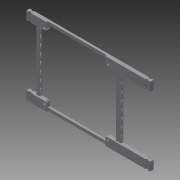
# Autodesk Inventor part: NUCholder
Saved by Autodesk Inventor 2015 (Build 190159000, 159)
## iProperties
Created: 2015-04-17
Part Number: NUCholder
Material: NylonD2W
Document SubType Name: Modeling
Designer: Akovo_000
Density: 0.93 g/cm^3
Appearance: Nylon 6
Mass: 13.1398 g
Surface Area: 149.789 cm^2
Volume: 14.1288 cm^3
Author: Akovo_000
Autodesk Inventor part; units mm, degrees
ref_plane "YZ Plane" through (0, 0, 0) normal (1, 0, 0) x (0, 1, 0)
ref_plane "XZ Plane" through (0, 0, 0) normal (0, 1, 0) x (-1, 0, 0)
ref_plane "XY Plane" through (0, 0, 0) normal (0, 0, 1) x (1, 0, 0)
sketch "Button Layer" plane through (0, 0, 0) normal (0, 1, 0) x (-1, 0, 0)
  line L0 (-73.3766, -28.1226) -> (16.7234, -28.1226)
  circle A0 centre (16.7234, -28.1226) radius 1.5
  circle A1 centre (-73.3766, -28.1226) radius 1.5
  line L1 (16.7234, 2.8734) -> (-73.3766, 2.8734)
  circle A2 centre (-11.2766, 30.8734) radius 28
  line L2 (-73.3766, 2.8734) -> (-73.3766, -28.1226)
  line L3 (-73.3766, 47.3774) -> (-73.3766, 2.8734)
  line L4 (16.7234, 2.8734) -> (16.7234, 58.8734)
  line L5 (16.7234, 2.8734) -> (16.7234, -28.1226)
  circle A3 centre (9.7234, -21.1226) radius 3
  circle A4 centre (9.7234, -21.1226) radius 2.5
  line L6 (9.7234, -21.1226) -> (16.7234, -21.1226)
  line L7 (16.7234, -21.1226) -> (16.7234, -28.1226)
  line L8 (16.7234, -28.1226) -> (9.7234, -28.1226)
  line L9 (9.7234, -28.1226) -> (9.7234, -21.1226)
  line L10 (9.7234, -21.1226) -> (-2.2766, -21.1226)
  line L11 (-2.2766, -21.1226) -> (-2.2766, -15.6226)
  line L12 (-2.2766, -15.6226) -> (9.7234, -15.6226)
  line L13 (9.7234, -15.6226) -> (9.7234, -21.1226)
  circle A5 centre (9.7234, -15.6226) radius 2.5
  circle A6 centre (-2.2766, -15.6226) radius 2.5
  line L14 (15.1646, -25.4226) -> (18.2823, -25.4226)
  line L15 (18.2823, -25.4226) -> (19.8411, -28.1226)
  line L16 (19.8411, -28.1226) -> (18.2823, -30.8226)
  line L17 (18.2823, -30.8226) -> (15.1646, -30.8226)
  line L18 (15.1646, -30.8226) -> (13.6057, -28.1226)
  line L19 (13.6057, -28.1226) -> (15.1646, -25.4226)
  line L20 (-74.9354, -25.4226) -> (-71.8177, -25.4226)
  line L21 (-71.8177, -25.4226) -> (-70.2589, -28.1226)
  line L22 (-70.2589, -28.1226) -> (-71.8177, -30.8226)
  line L23 (-71.8177, -30.8226) -> (-74.9354, -30.8226)
  line L24 (-74.9354, -30.8226) -> (-76.4943, -28.1226)
  line L25 (-76.4943, -28.1226) -> (-74.9354, -25.4226)
  line L26 (16.7234, 79.3734) -> (-73.3766, 79.3734)
  line L27 (-73.3766, -15.6266) -> (16.7234, -15.6266)
  circle A7 centre (16.7234, 79.3734) radius 1.5
  circle A8 centre (16.7234, -15.6266) radius 1.5
  circle A9 centre (-73.3766, -15.6266) radius 1.5
  circle A10 centre (-73.3766, 79.3734) radius 1.5
  line L28 (-73.3766, 59.8734) -> (16.7234, 59.8734)
  line L29 (-73.3766, 3.8734) -> (-73.3766, -15.6266)
  line L30 (-73.3766, 59.8734) -> (-73.3766, 79.3734)
  line L31 (-73.3766, 59.8734) -> (-73.3766, 3.8734)
  line L32 (16.7234, 3.8734) -> (16.7234, 59.8734)
  line L33 (16.7234, 3.8734) -> (16.7234, -15.6266)
  circle A11 centre (9.7234, -8.6266) radius 3
  circle A12 centre (9.7234, -8.6266) radius 2.5
  line L34 (9.7234, -8.6266) -> (16.7234, -8.6266)
  line L35 (16.7234, -8.6266) -> (16.7234, -15.6266)
  line L36 (16.7234, -15.6266) -> (9.7234, -15.6266)
  line L37 (9.7234, -15.6266) -> (9.7234, -8.6266)
  line L38 (9.7234, -8.6266) -> (-2.2766, -8.6266)
  line L39 (-2.2766, -8.6266) -> (-2.2766, -3.1266)
  line L40 (-2.2766, -3.1266) -> (9.7234, -3.1266)
  line L41 (9.7234, -3.1266) -> (9.7234, -8.6266)
  circle A13 centre (9.7234, -3.1266) radius 2.5
  circle A14 centre (-2.2766, -3.1266) radius 2.5
  line L42 (15.1646, -12.9266) -> (18.2823, -12.9266)
  line L43 (18.2823, -12.9266) -> (19.8411, -15.6266)
  line L44 (19.8411, -15.6266) -> (18.2823, -18.3266)
  line L45 (18.2823, -18.3266) -> (15.1646, -18.3266)
  line L46 (15.1646, -18.3266) -> (13.6057, -15.6266)
  line L47 (13.6057, -15.6266) -> (15.1646, -12.9266)
  line L48 (15.1646, 82.0734) -> (18.2823, 82.0734)
  line L49 (18.2823, 82.0734) -> (19.8411, 79.3734)
  line L50 (19.8411, 79.3734) -> (18.2823, 76.6734)
  line L51 (18.2823, 76.6734) -> (15.1646, 76.6734)
  line L52 (15.1646, 76.6734) -> (13.6057, 79.3734)
  line L53 (13.6057, 79.3734) -> (15.1646, 82.0734)
  line L54 (-74.9354, 82.0734) -> (-71.8177, 82.0734)
  line L55 (-71.8177, 82.0734) -> (-70.2589, 79.3734)
  line L56 (-70.2589, 79.3734) -> (-71.8177, 76.6734)
  line L57 (-71.8177, 76.6734) -> (-74.9354, 76.6734)
  line L58 (-74.9354, 76.6734) -> (-76.4943, 79.3734)
  line L59 (-76.4943, 79.3734) -> (-74.9354, 82.0734)
  line L60 (-74.9354, -12.9266) -> (-71.8177, -12.9266)
  line L61 (-71.8177, -12.9266) -> (-70.2589, -15.6266)
  line L62 (-70.2589, -15.6266) -> (-71.8177, -18.3266)
  line L63 (-71.8177, -18.3266) -> (-74.9354, -18.3266)
  line L64 (-74.9354, -18.3266) -> (-76.4943, -15.6266)
  line L65 (-76.4943, -15.6266) -> (-74.9354, -12.9266)
  line L66 (41.6234, -38.1226) -> (-138.3766, -38.1226)
  line L67 (-138.3766, -38.1226) -> (-138.3766, 63.8774)
  line L68 (-138.3766, 63.8774) -> (41.6234, 63.8774)
  line L69 (41.6234, 63.8774) -> (41.6234, -38.1226)
  circle A15 centre (-73.3766, -15.6266) radius 3.5
  circle A16 centre (16.7234, -15.6266) radius 3.5
  circle A17 centre (-73.3766, 79.3734) radius 3.5
  circle A18 centre (16.7234, 79.3734) radius 3.5
  line L70 (41.6234, -38.1226) -> (13.2234, -38.1226)
  line L71 (13.2234, -38.1226) -> (13.2234, -12.1266)
  line L72 (13.2234, -12.1266) -> (41.6234, -12.1266)
  line L73 (41.6234, -12.1266) -> (41.6234, -38.1226)
  line L74 (-138.3766, -38.1226) -> (-69.8766, -38.1226)
  line L75 (-69.8766, -38.1226) -> (-69.8766, -12.1266)
  line L76 (-69.8766, -12.1266) -> (-138.3766, -12.1266)
  line L77 (-138.3766, -12.1266) -> (-138.3766, -38.1226)
  line L78 (16.7234, 59.8734) -> (16.7234, 79.3734)
  point P0 (0, 0)
  point P1 (0, 0)
  point P2 (0, 0)
  dimension "d33" = 90.1
  dimension "d35" = 6
  dimension "d36" = 0.5
  dimension "d37" = 5
  dimension "d38" = 12
  dimension "d39" = 7
  dimension "d40" = 5.4
  dimension "d41" = 3
  dimension "d43" = 90.1
  dimension "d45" = 6
  dimension "d46" = 0.5
  dimension "d47" = 5
  dimension "d48" = 12
  dimension "d49" = 7
  dimension "d50" = 5.4
  dimension "d63" = 180
  dimension "d64" = 102
  dimension "d65" = 65
  dimension "d66" = 24.9
  dimension "d67" = 22.496
  dimension "d68" = 7
  dimension "d69" = 10
  dimension "d70" = 57
  constraints: 158 end point, 20 coincident, 19 centre point, 15 parallel, 10 perpendicular, 9 equal length, 9 horizontal, 8 equal radius, 8 tangent, 5 collinear, 4 vertical, 2 concentric, 78 other
  measures "d33" distance of L0.start L0.end
  measures "d35" diameter of A3
  measures "d36" radial gap between concentric circles of A3 A4
  measures "d37" diameter of A5
  measures "d38" distance between parallel lines of L11 L13
  measures "d39" distance of L6.start L6.end
  measures "d40" distance between parallel lines of L15 L18
  measures "d41" diameter of A7
  measures "d43" distance of L27.start L27.end
  measures "d45" diameter of A11
  measures "d46" radial gap between concentric circles of A11 A12
  measures "d47" diameter of A13
  measures "d48" distance between parallel lines of L39 L41
  measures "d49" distance of L34.start L34.end
  measures "d50" distance between parallel lines of L43 L46
  measures "d63" distance of L67.end L68.end
  measures "d64" distance of L66.end L67.end
  measures "d65" distance between parallel lines of L67 L29
  measures "d66" distance between parallel lines of L69 L32
  measures "d67" distance between parallel lines of L66 L27
  measures "d68" diameter of A15
  measures "d69" distance between parallel lines of L66 L0
  measures "d70" distance between parallel lines of L28 L1
sketch "NucSupport" plane through (0, 0, 0) normal (0, 1, 0) x (-1, 0, 0)
  line L0 (0, 0) -> (-175, 0)
  line L1 (-175, 0) -> (-175, 110)
  line L2 (-175, 110) -> (0, 110)
  line L3 (0, 110) -> (0, 0)
  line L4 (-24.9, 8.5) -> (-115, 8.5)
  line L5 (-115, 8.5) -> (-115, 101.5)
  line L6 (-115, 101.5) -> (-24.9, 101.5)
  line L7 (-24.9, 101.5) -> (-24.9, 8.5)
  line L8 (-24.9, 12) -> (0, 12)
  line L9 (-28.4, 8.5) -> (-28.4, 0)
  line L10 (-24.9, 98) -> (0, 98)
  line L11 (-28.4, 101.5) -> (-28.4, 110)
  line L12 (-111.5, 101.5) -> (-111.5, 110)
  line L13 (-115, 98) -> (-175, 98)
  line L14 (-115, 12) -> (-175, 12)
  line L15 (-111.5, 8.5) -> (-111.5, 0)
  circle A0 centre (-115, 8.5) radius 3.5
  circle A1 centre (-24.9, 8.5) radius 3.5
  circle A2 centre (-115, 101.5) radius 3.5
  circle A3 centre (-24.9, 101.5) radius 3.5
  dimension "d174" = 7
  dimension "d71" = 175
  dimension "d72" = 110
  dimension "d73" = 90.1
  dimension "d74" = 93
  dimension "d75" = 60
  dimension "d176" = 24.9
  dimension "d270" = 12
  constraints: 32 end point, 16 point on line, 9 equal length, 4 coincident, 4 horizontal, 2 horizontal alignment, 2 vertical, 2 vertical alignment, 1 perpendicular, 10 other
  measures "d71" distance of L0.start L0.end
  measures "d72" distance of L0.end L1.end
  measures "d73" distance of L5.end L6.end
  measures "d74" distance of L4.end L5.end
  measures "d75" distance between parallel lines of L1 L5
  measures "d176" distance between parallel lines of L3 L7
  measures "d270" distance between parallel lines of L13 L2
extrude "NucSupportHorizontal" add sketch "NucSupport" along normal blind 2 contours L0 L9 A1 L8 L3 | L0 L1 L14 A0 L15 | A1 L7 L4 | L4 L7 A1 | L10 A3 L11 L2 L3 | A0 L5 L4 | L4 L5 A0 | A3 L6 L7 | L7 L6 A3 | L1 L2 L12 A2 L13 | A2 L6 L5 | L5 L6 A2
sketch "Sketch4" plane through (0, 2, 0) normal (0, 1, 0) x (1, 0, 0)
  arc A0 (28.4, -101.5) -> (24.9, -98) centre (24.9, -101.5) ccw projected
  circle A1 centre (24.9, -101.5) radius 3.5
  arc A2 (115, -98) -> (111.5, -101.5) centre (115, -101.5) ccw projected
  circle A3 centre (115, -101.5) radius 3.5
  arc A4 (111.5, -8.5) -> (115, -12) centre (115, -8.5) ccw projected
  circle A5 centre (115, -8.5) radius 3.5
  arc A6 (24.9, -12) -> (28.4, -8.5) centre (24.9, -8.5) ccw projected
  circle A7 centre (24.9, -8.5) radius 3.5
  constraints: 7 equal radius, 4 centre point, 4 coincident
hole "Holes" at (24.9, 2, 101.5) at (24.9, 2, 8.5) at (115, 2, 8.5) at (115, 2, 101.5) direction (0, -1, 0) diameter 3.5 depth 7
sketch "Sketch6" plane through (0, 2, 0) normal (0, 1, 0) x (1, 0, 0)
  line L0 (0, 0) -> (28.4, 0)
  line L1 (28.4, 0) -> (28.4, -8.5)
  line L2 (28.4, -8.5) -> (28.4, 0) projected
  line L3 (24.9, -12) -> (0, -12)
  line L4 (0, -12) -> (0, 0)
  line L5 (0, 0) -> (0, -12) projected
  line L6 (0, -98) -> (24.9, -98)
  line L7 (24.9, -98) -> (0, -98) projected
  line L8 (0, -110) -> (28.4, -110) projected
  line L9 (28.4, -110) -> (0, -110)
  line L10 (0, -110) -> (0, -98)
  line L11 (111.5, -110) -> (111.5, -101.5)
  arc A0 (115, -98) -> (111.5, -101.5) centre (115, -101.5) ccw projected
  line L12 (115, -98) -> (175, -98)
  line L13 (175, -98) -> (115, -98) projected
  line L14 (175, -98) -> (175, -110)
  line L15 (175, -110) -> (111.5, -110)
  line L16 (111.5, 0) -> (175, 0)
  line L17 (175, 0) -> (111.5, 0) projected
  line L18 (175, 0) -> (175, -12)
  line L19 (175, -12) -> (115, -12)
  arc A1 (111.5, -8.5) -> (115, -12) centre (115, -8.5) ccw projected
  line L20 (111.5, -8.5) -> (111.5, 0)
  circle A2 centre (115, -101.5) radius 1.75 projected
  arc A3 (115, -98) -> (111.5, -101.5) centre (115, -101.5) ccw
  circle A4 centre (24.9, -8.5) radius 1.75 projected
  arc A5 (24.9, -12) -> (28.4, -8.5) centre (24.9, -8.5) ccw
  circle A6 centre (115, -8.5) radius 1.75 projected
  arc A7 (111.5, -8.5) -> (115, -12) centre (115, -8.5) ccw
  circle A8 centre (24.9, -101.5) radius 1.75 projected
  arc A9 (28.4, -101.5) -> (24.9, -98) centre (24.9, -101.5) ccw
  arc A10 (28.4, -101.5) -> (24.9, -98) centre (24.9, -101.5) ccw projected
  line L21 (28.4, -101.5) -> (28.4, -110)
  line L22 (0, -12) -> (24.9, -12) projected
  line L23 (28.4, -110) -> (28.4, -101.5) projected
  line L24 (111.5, -101.5) -> (111.5, -110) projected
  line L25 (111.5, 0) -> (111.5, -8.5) projected
  line L26 (16.9, -12) -> (16.9, -98)
  line L27 (11.9, -98) -> (11.9, -12)
  line L28 (125, -12) -> (125, -98)
  line L29 (175, -98) -> (115, -98) projected
  line L30 (115, -12) -> (175, -12) projected
  line L31 (132, -12) -> (132, -98)
  line L32 (28.4, 0) -> (111.5, 0)
  line L33 (111.5, 0) -> (111.5, -4.25)
  line L34 (111.5, -4.25) -> (28.4, -4.25)
  line L35 (28.4, -4.25) -> (28.4, 0)
  line L36 (111.5, -110) -> (28.4, -110)
  line L37 (28.4, -110) -> (28.4, -105.75)
  line L38 (28.4, -105.75) -> (111.5, -105.75)
  line L39 (111.5, -105.75) -> (111.5, -110)
  dimension "d179" = 5
  dimension "d181" = 7
  dimension "d183" = 8
  dimension "d184" = 10
  dimension "d269" = 12
  constraints: 56 end point, 9 perpendicular, 9 point on line, 8 point on circle, 7 parallel, 6 collinear, 5 tangent, 4 centre point, 4 coincident, 3 horizontal, 2 midpoint, 1 vertical
  measures "d179" distance between parallel lines of L27 L26
  measures "d181" distance between parallel lines of L31 L28
  measures "d183" distance from line of L26 A5.centre
  measures "d184" distance from line of A7.centre L28
  measures "d269" distance of L16.end L18.end
extrude "Big Holder" add sketch "Sketch6" along normal blind 3 contours L0 L1 A5 L3 L4 | L32 L20 L34 L1 | L16 L18 L19 A1 L20 | L3 L26 L6 L27 | L6 A9 L21 L8 L10 | L31 L12 L28 L19 | L12 L14 L15 L11 A0 | L21 L38 L11 L36
sketch "Air Grill" plane through (132, 2, 98) normal (1, 0, 0) x (0, 0, -1)
  line L0 (0, 3) -> (86, 3)
  line L1 (86, 3) -> (86, 0)
  line L2 (0, 0) -> (0, 3)
  line L3 (1, 3) -> (85, 3)
  line L4 (85, 3) -> (85, 2.5)
  line L5 (1, 2.5) -> (1, 3)
  line L6 (85, 0) -> (85, 0.5)
  line L7 (1, -1.5) -> (1, -2)
  line L8 (89.5, 3) -> (86, 3) projected
  line L9 (1, 2.5) -> (1, -1.5)
  line L10 (85, 2.5) -> (85, 0.5)
  line L11 (86, 0) -> (86, 3) projected
  line L12 (1, 2.5) -> (5.5566, 0.5)
  line L13 (1, 2.5) -> (5.9762, 2.5) construction
  line L14 (7.2983, 0.5) -> (10.0583, 2.5)
  line L15 (7.2983, 0.5) -> (10.7067, 0.5) construction
  line L16 (11.8, 2.5) -> (16.3566, 0.5)
  line L17 (18.0982, 0.5) -> (20.8583, 2.5)
  line L18 (18.0982, 0.5) -> (21.5067, 0.5) construction
  line L19 (22.5999, 2.5) -> (27.1565, 0.5)
  line L20 (28.8982, 0.5) -> (31.6582, 2.5)
  line L21 (28.8982, 0.5) -> (32.3067, 0.5) construction
  line L22 (33.3999, 2.5) -> (37.9565, 0.5)
  line L23 (33.3999, 2.5) -> (38.3761, 2.5) construction
  line L24 (39.6982, 0.5) -> (42.4582, 2.5)
  line L25 (11.8, 2.5) -> (9.0399, 0.5)
  line L26 (13.5416, 2.5) -> (18.0982, 0.5)
  line L27 (19.8399, 0.5) -> (22.5999, 2.5)
  line L28 (24.3416, 2.5) -> (28.8982, 0.5)
  line L29 (30.6399, 0.5) -> (33.3999, 2.5)
  line L30 (35.1416, 2.5) -> (39.6982, 0.5)
  line L31 (41.4398, 0.5) -> (44.1998, 2.5)
  line L32 (7.2983, 0.5) -> (5.5566, 0.5)
  line L33 (16.3566, 0.5) -> (18.0982, 0.5)
  line L34 (10.0583, 2.5) -> (11.8, 2.5)
  line L35 (11.8, 2.5) -> (11.8, 2.5)
  line L36 (13.5416, 2.5) -> (11.8, 2.5)
  line L37 (13.5416, 2.5) -> (20.8583, 2.5)
  line L38 (20.8583, 2.5) -> (22.5999, 2.5)
  line L39 (22.5999, 2.5) -> (22.5999, 2.5)
  line L40 (22.5999, 2.5) -> (24.3416, 2.5)
  line L41 (31.6582, 2.5) -> (24.3416, 2.5)
  line L42 (31.6582, 2.5) -> (33.3999, 2.5)
  line L43 (33.3999, 2.5) -> (33.3999, 2.5)
  line L44 (35.1416, 2.5) -> (33.3999, 2.5)
  line L45 (35.1416, 2.5) -> (42.4582, 2.5)
  line L46 (44.1998, 2.5) -> (42.4582, 2.5)
  line L47 (16.3566, 0.5) -> (9.0399, 0.5)
  line L48 (9.0399, 0.5) -> (7.2983, 0.5)
  line L49 (18.0982, 0.5) -> (19.8399, 0.5)
  line L50 (19.8399, 0.5) -> (27.1565, 0.5)
  line L51 (28.8982, 0.5) -> (27.1565, 0.5)
  line L52 (28.8982, 0.5) -> (30.6399, 0.5)
  line L53 (37.9565, 0.5) -> (30.6399, 0.5)
  line L54 (37.9565, 0.5) -> (39.6982, 0.5)
  line L55 (39.6982, 0.5) -> (41.4398, 0.5)
  line L56 (7.2983, 0.5) -> (2.7417, 2.5)
  line L57 (1, 2.5) -> (2.7417, 2.5)
  line L58 (10.0583, 2.5) -> (2.7417, 2.5)
  line L59 (5.5566, 0.5) -> (1, 0.5)
  line L60 (44.1998, 2.5) -> (48.7564, 0.5)
  line L61 (45.9415, 2.5) -> (50.4981, 0.5)
  line L62 (50.4981, 0.5) -> (53.2581, 2.5)
  line L63 (54.9998, 2.5) -> (59.5564, 0.5)
  line L64 (56.7415, 2.5) -> (61.2981, 0.5)
  line L65 (61.2981, 0.5) -> (64.0581, 2.5)
  line L66 (63.0398, 0.5) -> (65.7998, 2.5)
  line L67 (65.7998, 2.5) -> (70.3564, 0.5)
  line L68 (70.3564, 0.5) -> (72.098, 0.5)
  line L69 (98, -2) -> (98, 3) projected
  line L70 (72.098, 0.5) -> (74.8581, 2.5)
  line L71 (67.5414, 2.5) -> (72.098, 0.5)
  line L72 (72.098, 0.5) -> (73.8397, 0.5)
  line L73 (73.8397, 0.5) -> (76.5997, 2.5)
  line L74 (41.4398, 0.5) -> (48.7564, 0.5)
  line L75 (0, 3) -> (86, 3) projected
  line L76 (50.4981, 0.5) -> (48.7564, 0.5)
  line L77 (50.4981, 0.5) -> (52.2398, 0.5)
  line L78 (52.2398, 0.5) -> (59.5564, 0.5)
  line L79 (59.5564, 0.5) -> (61.2981, 0.5)
  line L80 (61.2981, 0.5) -> (63.0398, 0.5)
  line L81 (44.1998, 2.5) -> (45.9415, 2.5)
  line L82 (53.2581, 2.5) -> (45.9415, 2.5)
  line L83 (54.9998, 2.5) -> (56.7415, 2.5)
  line L84 (56.7415, 2.5) -> (64.0581, 2.5)
  line L85 (65.7998, 2.5) -> (64.0581, 2.5)
  line L86 (65.7998, 2.5) -> (67.5414, 2.5)
  line L87 (67.5414, 2.5) -> (74.8581, 2.5)
  line L88 (76.5997, 2.5) -> (74.8581, 2.5)
  line L89 (54.9998, 2.5) -> (52.2398, 0.5)
  line L90 (53.2581, 2.5) -> (54.9998, 2.5)
  line L91 (63.0398, 0.5) -> (70.3564, 0.5)
  line L92 (76.5997, 2.5) -> (81.1563, 0.5)
  line L93 (81.1563, 0.5) -> (82.898, 0.5)
  line L94 (86, 3) -> (0, 3) projected
  line L95 (82.898, 0.5) -> (78.3414, 2.5)
  line L96 (78.3414, 2.5) -> (76.5997, 2.5)
  line L97 (81.1563, 0.5) -> (73.8397, 0.5)
  line L98 (82.898, 0.5) -> (83.2583, 2.5)
  line L99 (83.2583, 2.5) -> (78.3414, 2.5)
  line L100 (0, 0) -> (86, 0) projected
  line L101 (83.2583, 2.5) -> (85, 2.5)
  line L102 (86, 0) -> (86, 3) projected
  line L103 (85, 2.5) -> (84.6397, 0.5)
  line L104 (82.898, 0.5) -> (84.6397, 0.5)
  line L105 (84.6397, 0.5) -> (85, 0.5)
  dimension "d185" = 1
  dimension "d186" = 1
  dimension "d198" = 0.7
  dimension "d201" = 0
  dimension "d272" = 0.5
  dimension "d273" = 0.5
  constraints: 198 end point, 44 collinear, 41 parallel, 28 horizontal, 6 point on line, 5 equal length, 5 perpendicular, 4 coincident, 1 midpoint, 1 vertical, 8 other
  measures "d185" distance between parallel lines of L2 L5
  measures "d186" distance between parallel lines of L1 L4
  measures "d198" distance between parallel lines of L56 L12
  measures "d201" distance of L17.start L26.end
  measures "d272" distance between parallel lines of L3 L84
  measures "d273" distance between parallel lines of L100 L97
extrude "Extrusion8" cut sketch "Air Grill" against normal blind 130 contours L12 L59 L9 | L10 L105 L103 | L58 L14 L56 | L98 L95 L99 | L25 L16 L47 | L97 L73 L92 | L37 L17 L26 | L70 L71 L87 | L27 L19 L50 | L91 L66 L67 | L41 L20 L28 | L65 L64 L84 | L29 L22 L53 | L78 L89 L63 | L45 L24 L30 | L62 L61 L82 | L31 L60 L74
sketch "Boss" plane through (0, 5, 0) normal (0, 1, 0) x (1, 0, 0)
  circle A0 centre (24.9, -101.5) radius 1.75 projected
  line L0 (23.3412, -98.8) -> (26.4588, -98.8)
  line L1 (26.4588, -98.8) -> (28.0177, -101.5)
  line L2 (28.0177, -101.5) -> (26.4588, -104.2)
  line L3 (26.4588, -104.2) -> (23.3412, -104.2)
  line L4 (23.3412, -104.2) -> (21.7823, -101.5)
  line L5 (21.7823, -101.5) -> (23.3412, -98.8)
  circle A1 centre (115, -101.5) radius 1.75 projected
  line L6 (116.5588, -98.8) -> (118.1177, -101.5)
  line L7 (118.1177, -101.5) -> (116.5588, -104.2)
  line L8 (116.5588, -104.2) -> (113.4412, -104.2)
  line L9 (113.4412, -104.2) -> (111.8823, -101.5)
  line L10 (111.8823, -101.5) -> (113.4412, -98.8)
  line L11 (113.4412, -98.8) -> (116.5588, -98.8)
  circle A2 centre (115, -8.5) radius 1.75 projected
  line L12 (116.5588, -5.8) -> (118.1177, -8.5)
  line L13 (118.1177, -8.5) -> (116.5588, -11.2)
  line L14 (116.5588, -11.2) -> (113.4412, -11.2)
  line L15 (113.4412, -11.2) -> (111.8823, -8.5)
  line L16 (111.8823, -8.5) -> (113.4412, -5.8)
  line L17 (113.4412, -5.8) -> (116.5588, -5.8)
  circle A3 centre (24.9, -8.5) radius 1.75 projected
  line L18 (26.4588, -5.8) -> (28.0177, -8.5)
  line L19 (28.0177, -8.5) -> (26.4588, -11.2)
  line L20 (26.4588, -11.2) -> (23.3412, -11.2)
  line L21 (23.3412, -11.2) -> (21.7823, -8.5)
  line L22 (21.7823, -8.5) -> (23.3412, -5.8)
  line L23 (23.3412, -5.8) -> (26.4588, -5.8)
  point P0 (0, 0)
  dimension "d232" = 5.4
  constraints: 48 end point, 4 coincident, 3 equal length, 3 parallel, 52 other
  measures "d232" distance between parallel lines of L1 L4
extrude "Extrusion10" cut sketch "Boss" against normal blind 2.4 contours A0 | L0 L1 L2 L3 L4 L5 | L6 L7 L8 L9 L10 L11 | L12 L13 L14 L15 L16 L17 | A3 | L18 L19 L20 L21 L22 L23
sketch "Sketch12" plane through (111.5, 0, 110) normal (0, 0, 1) x (1, 0, 0)
  line L0 (63.5, 0) -> (60.5, 0)
  line L1 (63.5, 5) -> (60.5, 5)
  line L2 (60.5, 0) -> (57.4, 0)
  line L3 (57.4, 0) -> (57.4, 1.25)
  line L4 (57.4, 1.25) -> (60.5, 1.25)
  line L5 (60.5, 1.25) -> (60.5, 0)
  line L6 (60.5, 5) -> (57.4, 5)
  line L7 (57.4, 5) -> (57.4, 3.75)
  line L8 (57.4, 3.75) -> (60.5, 3.75)
  line L9 (60.5, 3.75) -> (60.5, 5)
  line L10 (63.5, 0) -> (63.5, 5) projected
  line L11 (-111.5, 5) -> (-108.5, 5)
  line L12 (-108.5, 5) -> (-108.5, 3.75)
  line L13 (-108.5, 0) -> (-111.5, 0)
  line L14 (-111.5, 0) -> (-111.5, 5)
  line L15 (-108.5, 5) -> (-105.4, 5)
  line L16 (-105.4, 5) -> (-105.4, 3.75)
  line L17 (-105.4, 3.75) -> (-108.5, 3.75)
  line L18 (-108.5, 3.75) -> (-108.5, 5)
  line L19 (-108.5, 0) -> (-105.4, 0)
  line L20 (-105.4, 0) -> (-105.4, 1.25)
  line L21 (-105.4, 1.25) -> (-108.5, 1.25)
  line L22 (-108.5, 1.25) -> (-108.5, 0)
  line L23 (63.5, 0) -> (63.5, 5)
  line L24 (63.5, 0) -> (63.5, 5) projected
  line L25 (-108.5, 1.25) -> (-108.5, 0)
  line L26 (-108.5, 1.25) -> (-108.5, 2.5) construction
  line L27 (-108.5, 2.5) -> (-108.5, 3.75) construction
  line L28 (-111.5, 0) -> (-83.1, 0) projected
  dimension "d254" = 5
  dimension "d264" = 3
  dimension "d274" = 3
  dimension "d275" = 0
  dimension "d276" = 3.1
  constraints: 52 end point, 12 parallel, 9 equal length, 7 horizontal, 6 perpendicular, 2 collinear, 1 point on line, 1 vertical
  measures "d254" distance between parallel lines of L1 L0
  measures "d264" distance of L13.start L13.end
  measures "d274" distance between parallel lines of L9 L10
  measures "d275" distance between parallel lines of L28 L13
  measures "d276" distance between parallel lines of L20 L22
extrude "Attachment" cut sketch "Sketch12" against normal blind 1000
shell "Shell1" [suppressed]
body "Solid3"
